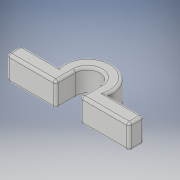
# Autodesk Inventor part: Motor hoop
Saved by Autodesk Inventor 2019 (Build 230136000, 136)
## iProperties
Created: 2021-03-23
Part Number: Motor hoop
Material: Generic
Document SubType Name: Modeling
Designer: User
Density: 1 g/cm^3
Appearance: Default
Author: User
Autodesk Inventor part; units mm, degrees
ref_plane "YZ Plane" through (0, 0, 0) normal (1, 0, 0) x (0, 1, 0)
ref_plane "XZ Plane" through (0, 0, 0) normal (0, 1, 0) x (-1, 0, 0)
ref_plane "XY Plane" through (0, 0, 0) normal (0, 0, 1) x (1, 0, 0)
sketch "Sketch1" plane through (0, 0, 0) normal (0, 1, 0) x (-1, 0, 0)
  arc A0 (-4.899, 1) -> (4.899, 1) centre (0, 0) ccw
  arc A1 (-2.5, 0) -> (2.5, 0) centre (0, 0) ccw
  line L0 (12.5, 1) -> (4.899, 1)
  line L1 (-4.899, 1) -> (-7, 1)
  line L2 (12.5, 1) -> (12.5, 4)
  line L3 (12.5, 4) -> (2.5, 4)
  line L4 (2.5, 4) -> (2.5, 0)
  line L5 (-2.5, 0) -> (-2.5, 4)
  line L6 (-2.5, 4) -> (-12.5, 4)
  line L7 (-12.5, 4) -> (-12.5, 1)
  line L8 (-12.5, 1) -> (-7, 1)
  dimension "d19" = 2.5
  dimension "d20" = 5
  dimension "d28" = 3
  dimension "d29" = 3
  dimension "d30" = 4
  dimension "d32" = 10
  dimension "d33" = 10
  constraints: 18 end point, 4 perpendicular, 4 point on circle, 2 centre point, 2 coincident, 2 horizontal, 2 point on line, 2 tangent, 1 parallel, 1 vertical
  measures "d19" radius of A1
  measures "d20" radius of A0
  measures "d28" distance between parallel lines of L0 L3
  measures "d29" distance between parallel lines of L3 L1
  measures "d30" distance from line of point (0, 0) L3
  measures "d32" distance between parallel lines of L2 L4
  measures "d33" distance between parallel lines of L5 L7
extrude "Extrusion1" add sketch "Sketch1" along normal mid plane 5
fillet "Fillet1" radius 0.5 4 edges at (0, 2.5, -2.5) (0, -2.5, -2.5) (0, -2.5, -5) (0, 2.5, -5)
fillet "Fillet1" radius 0.5 26 edges at (-2.5, 0, 4) (-2.5, 2.5, 2) (-2.5, -2.5, 2) (-12.5, 0, 4) (-7.5, 2.5, 4) (-7.5, -2.5, 4) (0, 2.5, -2.5) (0, -2.5, -2.5) (2.5, 2.5, 2) (7.5, 2.5, 4) (12.5, 2.5, 2.5) (8.6995, 2.5, 1) (0, 2.5, -5) (-8.6995, 2.5, 1) (-12.5, 2.5, 2.5) (-12.5, 0, 1) (-12.5, -2.5, 2.5) (2.5, 0, 4) (2.5, -2.5, 2) (7.5, -2.5, 4) (12.5, -2.5, 2.5) (8.6995, -2.5, 1) (0, -2.5, -5) (-8.6995, -2.5, 1) (12.5, 0, 1) (12.5, 0, 4)
body "Solid1"
